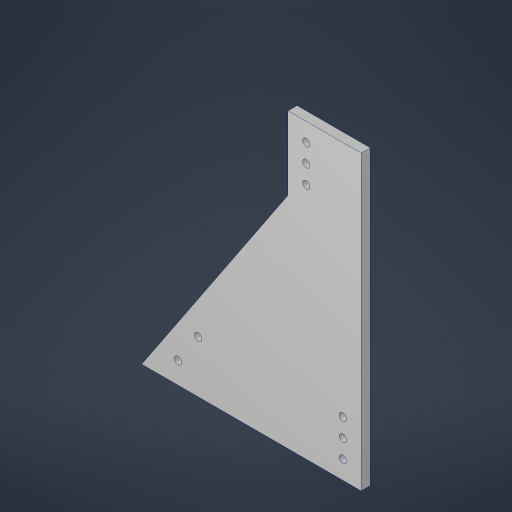
# Autodesk Inventor part: CL3-010
Saved by Autodesk Inventor 2023.4 (Build 274418000, 418)
## iProperties
RuleStatus: InUse
Created: 2025-01-31
Part Number: CL3-010
Material: Aluminum 6061
Document SubType Name: Modeling
Designer: brand
Mass: 132.735 g
Surface Area: 177.419 cm^2
Volume: 49.1612 cm^3
Density: 2.7 g/cm^3
Appearance: Aluminum - Flat
AfterDocNew0: SHOW
AfterDocOpen0: SHOW
Author: brand
Autodesk Inventor part; units mm, degrees
ref_plane "YZ Plane" through (0, 0, 0) normal (1, 0, 0) x (0, 1, 0)
ref_plane "XZ Plane" through (0, 0, 0) normal (0, 1, 0) x (-1, 0, 0)
ref_plane "XY Plane" through (0, 0, 0) normal (0, 0, 1) x (1, 0, 0)
sketch "Sketch1" plane through (0, 0, 0) normal (0, 0, 1) x (1, 0, 0)
  line L0 (-25.4, -101.6) -> (25.4, -101.6)
  line L1 (25.4, -101.6) -> (25.4, 101.6)
  line L2 (25.4, 101.6) -> (-25.4, 101.6)
  line L3 (-25.4, 101.6) -> (-25.4, -101.6)
  line L4 (-25.4, -101.6) -> (25.4, 101.6) construction
  line L5 (25.4, -101.6) -> (-25.4, 101.6) construction
  point P0 (0, 0)
  dimension "width" = 50.8
  dimension "length" = 203.2
  constraints: 12 end point, 2 midpoint, 2 parallel, 1 horizontal, 1 perpendicular
  measures "width" distance of L2.end L1.end
  measures "length" distance of L0.end L1.end
extrude "Extrusion1" add sketch "Sketch1" along normal mid plane 6.35
sketch "Sketch2" plane through (0, 0, 3.175) normal (0, 0, 1) x (1, 0, 0)
  line L0 (-25.4, -101.6) -> (-25.4, 101.6) construction
  line L1 (-25.4, 101.6) -> (25.4, 101.6) construction
  line L2 (25.4, 101.6) -> (25.4, -101.6) construction
  line L3 (25.4, -101.6) -> (-25.4, -101.6) construction
  point P0 (0, 0)
  point P1 (-12.7, 88.9)
  point P2 (-12.7, 76.2)
  point P3 (-12.7, 63.5)
  point P4 (12.7, -63.5)
  point P5 (12.7, -76.2)
  point P6 (12.7, -88.9)
  dimension "d4" = 25.4
  dimension "d5" = 12.7
  dimension "d6" = 12.7
  dimension "d7" = 12.7
  dimension "d8" = 12.7
  dimension "d9" = 12.7
  dimension "d10" = 12.7
  dimension "d11" = 25.4
  constraints: 4 vertical alignment
  measures "d4" distance from line of point (-12.7, 76.2) L1
  measures "d5" distance of point (-12.7, 76.2) point (-12.7, 88.9)
  measures "d6" distance of point (-12.7, 76.2) point (-12.7, 63.5)
  measures "d7" distance from line of L0 point (-12.7, 76.2)
  measures "d8" distance from line of L2 point (12.7, -76.2)
  measures "d9" distance of point (12.7, -63.5) point (12.7, -76.2)
  measures "d10" distance of point (12.7, -88.9) point (12.7, -76.2)
  measures "d11" distance from line of L3 point (12.7, -76.2)
hole "Hole1" at (-12.7, 88.9, 3.175) at (-12.7, 76.2, 3.175) at (-12.7, 63.5, 3.175) at (12.7, -63.5, 3.175) at (12.7, -76.2, 3.175) at (12.7, -88.9, 3.175) direction (0, 0, -1) diameter 5.1054 end through all clearance for "Flat Head Machine Screw (82)" size "#10" standard "Ansi Unified Screw Threads"
sketch "Sketch3" plane through (0, 0, 3.175) normal (0, 0, 1) x (1, 0, 0)
  circle A0 centre (12.7, -76.2) radius 2.5527 construction
  circle A1 centre (-12.7, 63.5) radius 2.5527 construction
  circle A2 centre (-12.7, 88.9) radius 2.5527 construction
  circle A3 centre (-12.7, 76.2) radius 2.5527 construction
  circle A4 centre (12.7, -63.5) radius 2.5527 construction
  circle A5 centre (12.7, -88.9) radius 2.5527 construction
  line L0 (-25.4, -101.6) -> (-25.4, 101.6) construction
  line L1 (-25.4, 101.6) -> (25.4, 101.6) construction
  line L2 (25.4, 101.6) -> (25.4, -101.6) construction
  line L3 (25.4, -101.6) -> (-25.4, -101.6) construction
  line L4 (-19.05, 95.25) -> (-19.05, -95.25) construction
  line L5 (-19.05, -95.25) -> (19.05, -95.25) construction
  line L6 (19.05, -95.25) -> (19.05, 95.25) construction
  line L7 (19.05, 95.25) -> (-19.05, 95.25) construction
  line L8 (-19.05, -95.25) -> (19.05, 95.25) construction
  line L9 (-19.05, 95.25) -> (19.05, -95.25) construction
  line L10 (-19.05, 0) -> (19.05, 0) construction
  line L11 (-19.05, -3.175) -> (19.05, -3.175) construction
  line L12 (-19.05, 3.175) -> (19.05, 3.175) construction
  circle A6 centre (-12.7, 63.5) radius 8.9027 construction
  circle A7 centre (-12.7, 76.2) radius 8.9027 construction
  circle A8 centre (-12.7, 88.9) radius 8.9027 construction
  circle A9 centre (12.7, -63.5) radius 8.9027 construction
  circle A10 centre (12.7, -76.2) radius 8.9027 construction
  circle A11 centre (12.7, -88.9) radius 8.9027 construction
  line L13 (3.7973, -63.5) -> (3.7973, -95.25) construction
  line L14 (12.7, -54.5973) -> (19.05, -54.5973) construction
  line L15 (-12.7, 54.5973) -> (-19.05, 54.5973) construction
  line L16 (-3.7973, 63.5) -> (-3.7973, 95.25) construction
  line L17 (15.8121, 95.25) -> (-19.05, -79.0606) construction
  line L18 (-15.8121, -95.25) -> (19.05, 79.0606) construction
  line L19 (-14.1573, 54.5973) -> (7.9555, -55.9669) construction
  line L20 (-7.9555, 55.9669) -> (14.1573, -54.5973) construction
  line L21 (-19.05, 54.5973) -> (-19.05, 3.175)
  line L22 (-19.05, 3.175) -> (-3.8729, 3.175)
  line L23 (-3.8729, 3.175) -> (-14.1573, 54.5973)
  line L24 (-14.1573, 54.5973) -> (-19.05, 54.5973)
  line L25 (3.8729, 3.175) -> (19.05, 3.175)
  line L26 (19.05, 3.175) -> (19.05, 79.0606)
  line L27 (19.05, 79.0606) -> (3.8729, 3.175)
  point P0 (0, 0)
  dimension "d19" = 6.35
  dimension "d20" = 3.175
  dimension "d21" = 3.175
  dimension "d22" = 6.35
  dimension "d23" = 6.35
  dimension "d24" = 6.35
  dimension "d25" = 6.35
  dimension "d26" = 6.35
  dimension "d27" = 6.35
  dimension "d28" = 3.175
  dimension "d29" = 3.175
  dimension "d30" = 3.175
  dimension "d31" = 3.175
  constraints: 48 end point, 23 point on line, 7 parallel, 6 centre point, 6 perpendicular, 6 point on circle, 4 tangent, 2 midpoint, 1 horizontal, 1 vertical, 3 other
  measures "d19" distance between parallel lines of L0 L4
  measures "d20" distance between parallel lines of L10 L11
  measures "d21" distance between parallel lines of L10 L12
  measures "d22" radial gap between concentric circles of A1 A6
  measures "d23" radial gap between concentric circles of A3 A7
  measures "d24" radial gap between concentric circles of A2 A8
  measures "d25" radial gap between concentric circles of A4 A9
  measures "d26" radial gap between concentric circles of A0 A10
  measures "d27" radial gap between concentric circles of A5 A11
  measures "d28" distance between parallel lines of L8 L17
  measures "d29" distance between parallel lines of L18 L8
  measures "d30" distance between parallel lines of L20 L9
  measures "d31" distance between parallel lines of L9 L19
sketch "Sketch4" plane through (0, 0, 3.175) normal (0, 0, 1) x (1, 0, 0)
  circle A0 centre (12.7, -76.2) radius 2.5527 construction
  circle A1 centre (-12.7, 63.5) radius 2.5527 construction
  circle A2 centre (-12.7, 88.9) radius 2.5527 construction
  circle A3 centre (-12.7, 76.2) radius 2.5527 construction
  circle A4 centre (12.7, -63.5) radius 2.5527 construction
  circle A5 centre (12.7, -88.9) radius 2.5527 construction
  line L0 (-25.4, -101.6) -> (-25.4, 101.6) construction
  line L1 (-25.4, 101.6) -> (25.4, 101.6) construction
  line L2 (25.4, 101.6) -> (25.4, -101.6) construction
  line L3 (25.4, -101.6) -> (-25.4, -101.6) construction
  line L4 (25.4, -101.6) -> (-127, -101.6) construction
  line L5 (-127, -101.6) -> (-127, -50.8) construction
  line L6 (-127, -50.8) -> (25.4, -50.8) construction
  line L7 (25.4, -50.8) -> (25.4, -101.6) construction
  line L8 (-127, -101.6) -> (-25.4, -101.6)
  line L9 (-25.4, -101.6) -> (-25.4, 101.6)
  line L10 (-25.4, 50.8) -> (-127, -101.6)
  circle A6 centre (-101.8479, -86.767) radius 4.7625 construction
  circle A7 centre (-87.7585, -65.633) radius 4.7625 construction
  line L11 (-101.8479, -86.767) -> (-87.7585, -65.633) construction
  point P0 (0, 0)
  point P1 (-127, -76.2)
  point P2 (-94.8032, -76.2)
  dimension "d32" = 50.8
  dimension "d33" = 152.4
  dimension "d36" = 9.525
  dimension "d37" = 9.525
  dimension "d38" = 12.7
  dimension "d39" = 25.4
  dimension "d47" = 50.8
  constraints: 16 end point, 3 parallel, 2 centre point, 2 horizontal, 2 midpoint, 2 perpendicular, 1 horizontal alignment, 1 point on line
  measures "d32" distance of L4.end L5.end
  measures "d33" distance between parallel lines of L2 L5
  measures "d36" diameter of A6
  measures "d37" diameter of A7
  measures "d38" distance between parallel lines of L10 L11
  measures "d39" distance of L11.start L11.end
  measures "d47" distance from line of L1 L10.start
extrude "Extrusion2" add sketch "Sketch4" against normal up to surface (6.35 mm away)
sketch "Sketch5" plane through (0, 0, 3.175) normal (0, 0, 1) x (1, 0, 0)
  point P0 (0, 0)
  point P1 (-87.7585, -65.633)
  point P2 (-101.8479, -86.767)
hole "Hole2" at (-87.7585, -65.633, 3.175) at (-101.8479, -86.767, 3.175) direction (0, 0, -1) diameter 5.1054 end through all clearance for "Flat Head Machine Screw (82)" size "#10" standard "Ansi Unified Screw Threads"
equation "\"d6\" = d5"
equation "\"d8\" = d7"
equation "\"d9\" = d5"
equation "\"d10\" = d9"
equation "\"d11\" = d4"
equation "\"d20\" = 0.5 * d19"
equation "\"d21\" = d20"
equation "\"d22\" = d19"
equation "\"d23\" = d19"
equation "\"d24\" = d19"
equation "\"d25\" = d19"
equation "\"d26\" = d19"
equation "\"d27\" = d19"
equation "\"d28\" = d21"
equation "\"d29\" = d28"
equation "\"d30\" = d20"
equation "\"d31\" = d30"
equation "\"d37\" = d36"
body "Solid1"
